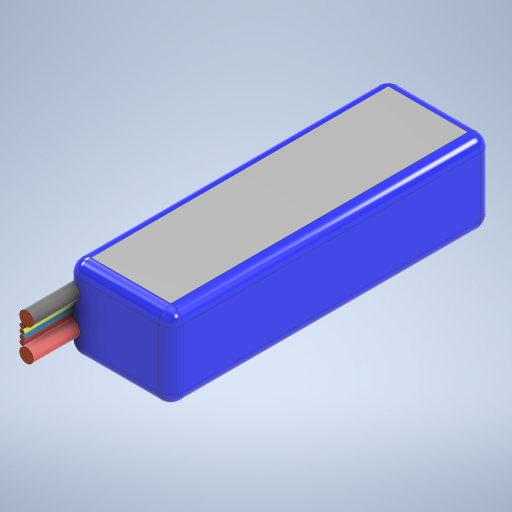
# Autodesk Inventor part: Аккамулятор
Saved by Autodesk Inventor 2023 (Build 270158000, 158)
## iProperties
Created: 2022-12-23
Part Number: Аккамулятор
Material: Типовые
Document SubType Name: Modeling
Designer: Khasal
Density: 1 g/cm^3
Appearance: По умолчанию
Author: Khasal
Autodesk Inventor part; units mm, degrees
ref_plane "YZ Plane" through (0, 0, 0) normal (1, 0, 0) x (0, 1, 0)
ref_plane "XZ Plane" through (0, 0, 0) normal (0, 1, 0) x (-1, 0, 0)
ref_plane "XY Plane" through (0, 0, 0) normal (0, 0, 1) x (1, 0, 0)
sketch "Эскиз1" plane through (0, 0, 0) normal (0, 1, 0) x (-1, 0, 0)
  line L0 (17, -52.5) -> (-17, -52.5)
  line L1 (-17, -52.5) -> (-17, 52.5)
  line L2 (-17, 52.5) -> (17, 52.5)
  line L3 (17, 52.5) -> (17, -52.5)
  line L4 (17, -52.5) -> (-17, 52.5) construction
  line L5 (-17, -52.5) -> (17, 52.5) construction
  point P0 (0, 0)
  dimension "d0" = 105
  dimension "d1" = 34
  constraints: 12 end point, 2 midpoint, 2 parallel, 1 horizontal, 1 perpendicular
  measures "d0" distance of L2.end L0.start
  measures "d1" distance of L0.start L0.end
extrude "Выдавливание1" add sketch "Эскиз1" along normal blind 27
fillet "Сопряжение1" radius 4 12 edges at (17, 0, 0) (-17, 0, 0) (-17, 27, 0) (17, 27, 0) (0, 27, 52.5) (17, 13.5, 52.5) (0, 0, 52.5) (-17, 13.5, 52.5) (17, 13.5, -52.5) (0, 0, -52.5) (-17, 13.5, -52.5) (0, 27, -52.5)
sketch "Эскиз2" plane through (-13, 4, 52.5) normal (0, 0, 1) x (1, 0, 0)
  line L0 (26, 23) -> (0, 23) projected
  circle A0 centre (-1.8428, 14.4631) radius 2.25
  circle A1 centre (-1.8428, 4.066) radius 2.25
  circle A2 centre (-3.2811, 6.8739) radius 0.75
  circle A3 centre (-3.2811, 8.3904) radius 0.75
  circle A4 centre (-3.2811, 10.0466) radius 0.75
  circle A5 centre (-3.2811, 11.6568) radius 0.75
  point P0 (13, -4)
  dimension "d5" = 4.5
  dimension "d6" = 4.5
  dimension "d7" = 1.5
  dimension "d8" = 1.5
  dimension "d9" = 1.5
  dimension "d10" = 1.5
  constraints: 6 centre point
  measures "d5" diameter of A0
  measures "d6" diameter of A1
  measures "d7" diameter of A2
  measures "d8" diameter of A3
  measures "d9" diameter of A4
  measures "d10" diameter of A5
extrude "Выдавливание2" add sketch "Эскиз2" along normal blind 15.25 and the other way blind 4
